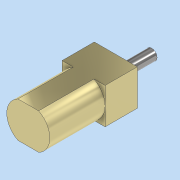
# Autodesk Inventor part: 모터
Saved by Autodesk Inventor 2020 (Build 240168000, 168)
## iProperties
Created: 2020-05-03
Part Number: 모터
Material: 일반
Document SubType Name: Modeling
Designer: sbahn
Density: 1 g/cm^3
Appearance: 기본값
Author: sbahn
Autodesk Inventor part; units mm, degrees
ref_plane "YZ Plane" through (0, 0, 0) normal (1, 0, 0) x (0, 1, 0)
ref_plane "XZ Plane" through (0, 0, 0) normal (0, 1, 0) x (-1, 0, 0)
ref_plane "XY Plane" through (0, 0, 0) normal (0, 0, 1) x (1, 0, 0)
sketch "스케치1" plane through (0, 0, 0) normal (0, 0, 1) x (1, 0, 0)
  line L0 (-6, 5) -> (6, 5)
  line L1 (6, 5) -> (6, -5)
  line L2 (6, -5) -> (-6, -5)
  line L3 (-6, -5) -> (-6, 5)
  line L4 (-6, 5) -> (6, -5) construction
  line L5 (6, 5) -> (-6, -5) construction
  point P0 (0, 0)
  dimension "d0" = 12
  dimension "d1" = 10
  constraints: 12 end point, 2 midpoint, 2 parallel, 1 horizontal, 1 perpendicular
  measures "d0" distance of L1.end L2.end
  measures "d1" distance of L0.end L1.end
extrude "돌출1" add sketch "스케치1" along normal blind 9
sketch "스케치2" plane through (0, 0, 9) normal (0, 0, 1) x (1, 0, 0)
  line L0 (-6, 5) -> (-6, -5) projected
  line L1 (-6, -5) -> (6, -5) projected
  line L2 (6, -5) -> (6, 5) projected
  line L3 (6, 5) -> (-6, 5) projected
  line L4 (-2.8796, -5) -> (2.8796, -5)
  line L5 (2.8796, -5) -> (2.8796, 5) construction
  line L6 (2.8796, 5) -> (-2.8796, 5)
  line L7 (-2.8796, 5) -> (-2.8796, -5) construction
  line L8 (-2.8796, -5) -> (2.8796, 5) construction
  line L9 (2.8796, -5) -> (-2.8796, 5) construction
  line L10 (-6, 0) -> (6, 0) construction
  arc A0 (-2.8796, 5) -> (-2.8796, -5) centre (-0.4339, 0) ccw
  arc A1 (2.8796, -5) -> (2.8796, 5) centre (0.4339, 0) ccw
  point P0 (0, 0)
  constraints: 14 end point, 6 point on circle, 4 midpoint, 2 centre point, 2 parallel, 1 horizontal, 1 perpendicular, 1 point on line
extrude "돌출2" add sketch "스케치2" along normal blind 15.4 contours A0 L3 A1 L1
sketch "스케치3" plane through (0, 0, 0) normal (0, 0, -1) x (-1, 0, 0)
  circle A0 centre (0, 0) radius 2
  dimension "d6" = 4
  constraints: 1 centre point, 1 coincident
  measures "d6" diameter of A0
extrude "돌출3" add sketch "스케치3" along normal blind 0.8
sketch "스케치4" plane through (0, 0, 0) normal (0, 0, -1) x (-1, 0, 0)
  circle A0 centre (0, 0) radius 1.5
  dimension "d9" = 3
  constraints: 1 centre point, 1 coincident
  measures "d9" diameter of A0
extrude "돌출4" add sketch "스케치4" along normal blind 10
